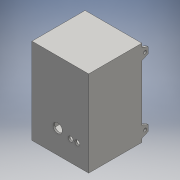
# Autodesk Inventor part: Housing for Filter
Saved by Autodesk Inventor 2016 (Build 200138000, 138)
## iProperties
Created: 2018-01-17
Part Number: Housing for Filter
Material: Generic
Document SubType Name: Modeling
Designer: trevo
Density: 1 g/cm^3
Appearance: Default
Author: trevo
Autodesk Inventor part; units mm, degrees
ref_plane "YZ Plane" through (0, 0, 0) normal (1, 0, 0) x (0, 1, 0)
ref_plane "XZ Plane" through (0, 0, 0) normal (0, 1, 0) x (-1, 0, 0)
ref_plane "XY Plane" through (0, 0, 0) normal (0, 0, 1) x (1, 0, 0)
sketch "Sketch1" plane through (0, 0, 0) normal (0, 1, 0) x (-1, 0, 0)
  line L0 (0, 0) -> (-64, 0)
  line L1 (-64, 0) -> (-64, -97)
  line L2 (-64, -97) -> (0, -97)
  line L3 (0, -97) -> (0, 0)
  dimension "d1" = 64
  dimension "d2" = 97
  constraints: 8 end point, 2 parallel, 1 horizontal, 1 perpendicular
  measures "d1" distance of L0.start L0.end
  measures "d2" distance of L2.end L0.start
extrude "Extrusion1" add sketch "Sketch1" along normal blind 60
shell "Shell1" thickness 2 removed faces 1 at (21.3333, 60, -64.6667)
sketch "Sketch2" plane through (2, 2, -2) normal (0, 1, 0) x (1, 0, 0)
  line L0 (60, 93) -> (0, 93) projected
  line L1 (30, 93) -> (30, 0) construction
  line L2 (60, 0) -> (0, 0) projected
  line L3 (0, 0) -> (0, 93) projected
  line L4 (0, 46.5) -> (60, 46.5) construction
  line L5 (60, 0) -> (60, 93) projected
  circle A0 centre (6.8, 79.9) radius 3
  circle A1 centre (6.8, 79.9) radius 1.75
  circle A2 centre (53.2, 79.9) radius 3
  circle A3 centre (53.2, 79.9) radius 1.75
  circle A4 centre (6.8, 13.1) radius 3
  circle A5 centre (6.8, 13.1) radius 1.75
  circle A6 centre (53.2, 13.1) radius 3
  circle A7 centre (53.2, 13.1) radius 1.75
  point P0 (-2, -2)
  dimension "d6" = 6
  dimension "d7" = 1.25
  dimension "d8" = 23.2
  dimension "d9" = 33.4
  constraints: 8 centre point, 6 symmetric about line, 4 coincident, 4 end point, 4 midpoint, 6 other
  measures "d6" diameter of A0
  measures "d7" radial gap between concentric circles of A0 A1
  measures "d8" distance from line of L1 A0.centre
  measures "d9" distance from line of L4 A0.centre
extrude "Extrusion2" add sketch "Sketch2" along normal blind 6 contours A0 | A2 | A4 | A6
sketch "Sketch3" plane through (2, 2, -2) normal (0, 1, 0) x (1, 0, 0)
  circle A0 centre (53.2, 79.9) radius 1.75 projected
  circle A1 centre (27, 68.41) radius 5.25
  circle A2 centre (41.72, 71.77) radius 2.75
  circle A3 centre (49.23, 71.77) radius 2.75
  point P0 (-2, -2)
  dimension "d12" = 11.49
  dimension "d13" = 26.2
  dimension "d14" = 10.5
  dimension "d15" = 0
  dimension "d16" = 5.5
  dimension "d17" = 5.5
  dimension "d18" = 3.97
  dimension "d19" = 8.13
  dimension "d20" = 7.51
  constraints: 3 centre point
  measures "d12" vertical distance of A0.centre A1.centre
  measures "d13" horizontal distance of A0.centre A1.centre
  measures "d14" diameter of A1
  measures "d15" vertical distance of A2.centre A3.centre
  measures "d16" diameter of A2
  measures "d17" diameter of A3
  measures "d18" horizontal distance of A3.centre A0.centre
  measures "d19" vertical distance of A3.centre A0.centre
  measures "d20" distance of A3.centre A2.centre
extrude "Extrusion3" cut sketch "Sketch3" against normal through all contours A1 | A2 | A3
sketch "Sketch4" plane through (64, 0, 0) normal (1, 0, 0) x (0, 0, -1)
  line L0 (0, 0) -> (97, 0) projected
  line L1 (48.5, 0) -> (48.5, 60) construction
  line L2 (95, 60) -> (2, 60) projected
  line L3 (4, 60) -> (17, 60)
  line L4 (14, 67) -> (7, 67)
  line L5 (0, 0) -> (0, 60) projected
  line L6 (4, 60) -> (7, 67)
  line L7 (17, 60) -> (14, 67)
  circle A0 centre (10.5, 63.5) radius 1.75
  line L8 (83, 67) -> (90, 67)
  line L9 (93, 60) -> (90, 67)
  line L10 (80, 60) -> (83, 67)
  circle A1 centre (86.5, 63.5) radius 1.75
  line L11 (80, 60) -> (93, 60)
  dimension "d28" = 7
  dimension "d29" = 4
  dimension "d30" = 13
  dimension "d31" = 7
  dimension "d32" = 3
  dimension "d33" = 3.5
  dimension "d34" = 3.5
  dimension "d35" = 6.5
  constraints: 18 end point, 5 symmetric about line, 2 centre point, 2 midpoint, 1 collinear, 1 horizontal, 1 parallel, 1 point on line, 1 other
  measures "d28" distance between parallel lines of L2 L4
  measures "d29" distance of L3.start L5.end
  measures "d30" distance of L3.end L3.start
  measures "d31" distance of L4.end L4.start
  measures "d32" horizontal distance of L4.end L3.start
  measures "d33" diameter of A0
  measures "d34" distance from line of L4 A0.centre
  measures "d35" horizontal distance of L3.start A0.centre
extrude "Extrusion4" add sketch "Sketch4" against normal blind 64
sketch "Sketch5" plane through (0, 60, 0) normal (0, 1, 0) x (1, 0, 0)
  line L0 (62, 2) -> (2, 2) projected
  line L1 (2, 93) -> (2, 95) projected
  line L2 (62, 2) -> (2, 2)
  line L3 (2, 2) -> (2, 95)
  line L4 (2, 95) -> (62, 95)
  line L5 (62, 95) -> (62, 2)
  point P0 (0, 0)
  constraints: 8 end point, 2 parallel, 1 horizontal, 1 perpendicular
extrude "Extrusion5" cut sketch "Sketch5" along normal through all
sketch "Sketch6" plane through (0, 0, -97) normal (-1, 0, 0) x (0, 0, 1)
  line L0 (2, 2) -> (2, 60) projected
  line L1 (17, 60) -> (80, 60) projected
  line L2 (85.5, 49.8) -> (73.5, 49.8)
  line L3 (73.5, 49.8) -> (73.5, 42.3)
  line L4 (73.5, 42.3) -> (85.5, 42.3)
  line L5 (85.5, 42.3) -> (85.5, 49.8)
  line L6 (97, 0) -> (97, 60) projected
  dimension "d48" = 7.5
  dimension "d49" = 10.2
  dimension "d51" = 11.5
  dimension "d52" = 23.5
  constraints: 8 end point, 2 parallel, 1 horizontal, 1 perpendicular
  measures "d48" distance of L4.end L2.start
  measures "d49" distance between parallel lines of L1 L2
  measures "d51" distance between parallel lines of L6 L5
  measures "d52" distance between parallel lines of L6 L3
extrude "Extrusion6" cut sketch "Sketch6" against normal up to next
body "Solid1"
